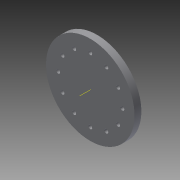
# Autodesk Inventor part: bay container 12 bottom
Saved by Autodesk Inventor 2015 (Build 190159000, 159)
## iProperties
Created: 2014-10-01
Part Number: bay container 12 bottom
Material: Generic
Document SubType Name: Modeling
Designer: ericd_000
Density: 1 g/cm^3
Appearance: Default
Author: ericd_000
Autodesk Inventor part; units mm, degrees
ref_plane "YZ Plane" through (0, 0, 0) normal (1, 0, 0) x (0, 1, 0)
ref_plane "XZ Plane" through (0, 0, 0) normal (0, 1, 0) x (-1, 0, 0)
ref_plane "XY Plane" through (0, 0, 0) normal (0, 0, 1) x (1, 0, 0)
sketch "Sketch1" plane through (0, 0, 0) normal (0, 1, 0) x (-1, 0, 0)
  circle A0 centre (0, 0) radius 45.5
  dimension "d0" = 91
  constraints: 1 centre point, 1 coincident
  measures "d0" diameter of A0
extrude "Extrusion1" add sketch "Sketch1" along normal blind 7
sketch "Sketch5" plane through (0, 7, 0) normal (0, 1, 0) x (1, 0, 0)
  circle A0 centre (0, 0) radius 6
  dimension "d27" = 12
  constraints: 1 centre point, 1 coincident
  measures "d27" diameter of A0
extrude "Extrusion5" add sketch "Sketch5" along normal blind 2
sketch "Sketch7" plane through (0, 0, 0) normal (0, -1, 0) x (1, 0, 0)
  circle A0 centre (0, 0) radius 45.5 projected
  line L0 (0, 0) -> (33, 0)
  circle A1 centre (33, 0) radius 2
  dimension "d37" = 4
  dimension "d38" = 33
  constraints: 2 end point, 1 centre point, 1 coincident, 1 horizontal
  measures "d37" diameter of A1
  measures "d38" distance of L0.start L0.end
extrude "Extrusion7" cut sketch "Sketch7" against normal blind 10 contours A1
pattern_circular "Circular Pattern1" count 12 over 360 about axis through (0, 0, 0) along (0, -1, 0) of "Extrusion7"
body "Solid1"
